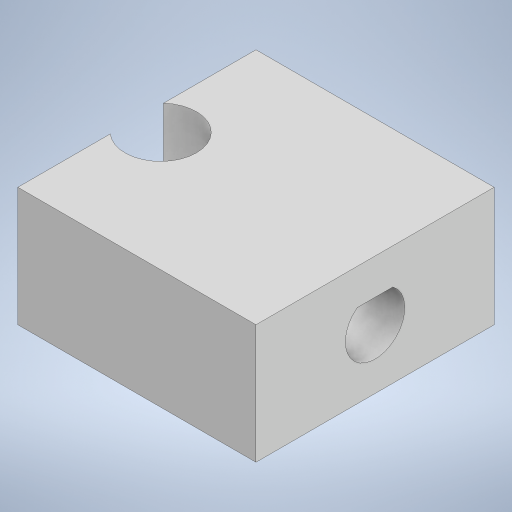
# Autodesk Inventor part: LazerMount
Saved by Autodesk Inventor 2024 (Build 280153000, 153)
## iProperties
Created: 2025-05-07
Part Number: LazerMount
Material: Generic
Document SubType Name: Modeling
Designer: Bjarni Heselmans
Density: 1 g/cm^3
Appearance: Default
Author: Bjarni Heselmans
Autodesk Inventor part; units mm, degrees
ref_plane "YZ Plane" through (0, 0, 0) normal (1, 0, 0) x (0, 1, 0)
ref_plane "XZ Plane" through (0, 0, 0) normal (0, 1, 0) x (-1, 0, 0)
ref_plane "XY Plane" through (0, 0, 0) normal (0, 0, 1) x (1, 0, 0)
sketch "Sketch1" plane through (0, 0, 0) normal (0, 0, 1) x (1, 0, 0)
  arc A0 (-2, -2.2361) -> (-2, 2.2361) centre (0, 0) ccw
  line L0 (-3, 0) -> (-2, 0)
  line L1 (-2, 0) -> (-2, 2.2361)
  line L2 (-2, 2.2361) -> (-2, -2.2361)
  line L3 (3, 0) -> (18, 0)
  line L4 (18, 0) -> (18, 10)
  line L5 (18, 10) -> (-2, 10)
  line L6 (-2, 10) -> (-2, 0)
  line L7 (3, 0) -> (18, 0)
  line L8 (18, 0) -> (18, -10)
  line L9 (18, -10) -> (-2, -10)
  line L10 (-2, -10) -> (-2, 0)
  point P0 (-2, 2.2361)
  point P1 (-2, -2.2361)
  dimension "d0" = 6
  dimension "d1" = 1
  dimension "d2" = 20
  dimension "d3" = 10
  dimension "d4" = 10
  constraints: 22 end point, 4 parallel, 3 horizontal, 3 perpendicular, 3 point on circle, 1 centre point, 1 coincident, 1 point on line
  measures "d0" diameter of A0
  measures "d1" distance of L0.start L0.end
  measures "d2" distance of L5.end L4.end
  measures "d3" distance of L4.end L3.end
  measures "d4" distance of L7.end L8.end
sketch "Sketch2" plane through (0, 0, 0) normal (0, 0, 1) x (1, 0, 0)
  point P0 (0, 0)
extrude "Extrusion1" add sketch "Sketch1" along normal blind 10 contours A0 L3 L8 L9 L10 | A0 L6 L5 L4 L3
sketch "Sketch3" plane through (18, -10, 0) normal (1, 0, 0) x (0, 0, -1)
  line L0 (0, 0) -> (-10, 0) projected
  line L1 (-10, 20) -> (-10, 12.2361) projected
  line L2 (0, 0) -> (-10, 0)
  line L3 (-10, 0) -> (-10, 20)
  line L4 (-10, 20) -> (0, 20)
  line L5 (0, 20) -> (0, 0)
  arc A0 (-7, 8.5) -> (-7, 11.5) centre (-5, 10) ccw
  line L6 (-7.5, 10) -> (-7, 10)
  line L7 (-7, 11.5) -> (-7, 8.5)
  point P0 (0, 10)
  dimension "d7" = 5
  dimension "d8" = 0.5
  constraints: 12 end point, 2 horizontal, 2 parallel, 2 point on circle, 1 centre point, 1 perpendicular, 1 vertical
  measures "d7" diameter of A0
  measures "d8" distance of L6.start L6.end
extrude "Extrusion2" cut sketch "Sketch3" against normal blind 12 contours L7 A0
body "Solid1"
